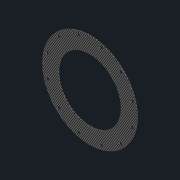
# Autodesk Inventor part: unit-plate3
Saved by Autodesk Inventor 2021 (Build 250183000, 183)
## iProperties
Created: 2021-07-12
Part Number: unit-plate3
Material: CFRP
Document SubType Name: Sheet Metal
Designer: yuta0
Density: 1.43 g/cm^3
Sheet Metal Rule: Default_mm
Appearance: カーボンファイバー
Mass: 9.12373 g
Surface Area: 136.539 cm^2
Volume: 6.38023 cm^3
Author: yuta0
Autodesk Inventor part; units mm, degrees
ref_plane "YZ Plane" through (0, 0, 0) normal (1, 0, 0) x (0, 1, 0)
ref_plane "XZ Plane" through (0, 0, 0) normal (0, 1, 0) x (-1, 0, 0)
ref_plane "XY Plane" through (0, 0, 0) normal (0, 0, 1) x (1, 0, 0)
sketch "スケッチ4" plane through (0, 0, 1) normal (0, 0, 1) x (1, 0, 0)
  circle A0 centre (16.1762, 60.3704) radius 2.25 projected
  circle A1 centre (-16.1762, 60.3704) radius 2.25 projected
  circle A2 centre (0, 0) radius 67.5 projected
  circle A3 centre (-16.1762, 60.3704) radius 5
  circle A4 centre (16.1762, 60.3704) radius 5
  circle A5 centre (0, 0) radius 62.5
  point P0 (-11.2987, 61.4702)
  point P1 (11.2987, 61.4702)
  point P2 (17.4703, 65.2)
  point P3 (-17.4703, 65.2)
  constraints: 2 centre point, 2 tangent, 3 other
sketch "スケッチ1" plane through (0, 0, 0) normal (0, 0, 1) x (1, 0, 0)
  circle A0 centre (0, 0) radius 67.5
  dimension "d0" = 135
  measures "d0" diameter of A0
extrude "プレート1" add sketch "スケッチ1" along normal blind 1
sketch "スケッチ2" plane through (0, 0, 1) normal (0, 0, 1) x (1, 0, 0)
  circle A0 centre (0, 0) radius 44.5
  dimension "d2" = 89
  constraints: 1 centre point, 1 coincident
  measures "d2" diameter of A0
extrude "押し出し1" cut sketch "スケッチ2" against normal through all
sketch "スケッチ3" plane through (0, 0, 1) normal (0, 0, 1) x (1, 0, 0)
  circle A0 centre (0, 0) radius 62.5
  point P0 (16.1762, 60.3704)
  point P1 (-16.1762, 60.3704)
  point P2 (-44.1942, 44.1942)
  point P3 (-60.3704, 16.1762)
  point P4 (-60.3704, -16.1762)
  point P5 (-44.1942, -44.1942)
  point P6 (-16.1762, -60.3704)
  point P7 (16.1762, -60.3704)
  point P8 (44.1942, -44.1942)
  point P9 (60.3704, -16.1762)
  point P10 (60.3704, 16.1762)
  point P11 (44.1942, 44.1942)
  dimension "d5" = 125
  dimension "d8" = 360
  dimension "d23" = 0
  constraints: 1 coincident, 16 other
  measures "d23" vertical distance of point (-16.176, 60.37) point (16.176, 60.37)
hole "穴1" at (16.1762, 60.3704, 1) at (-16.1762, 60.3704, 1) at (-44.1942, 44.1942, 1) at (-60.3704, 16.1762, 1) at (-60.3704, -16.1762, 1) at (-44.1942, -44.1942, 1) at (-16.1762, -60.3704, 1) at (16.1762, -60.3704, 1) at (44.1942, -44.1942, 1) at (60.3704, -16.1762, 1) at (60.3704, 16.1762, 1) at (44.1942, 44.1942, 1) direction (0, 0, -1) diameter 4.5 end through all clearance for "Flat Head Machine Screw" size "M4" standard "Ansi Metric M Profile"
equation "\"d15\" = Thickness"
equation "\"d1\" = Thickness"
equation "\"BendRadius\" = Thickness"
equation "\"BendReliefWidth\" = Thickness"
equation "\"BendReliefDepth\" = 0.5 * Thickness"
equation "\"CornerReliefSize\" = 4 * Thickness"
equation "\"MinimumRemnant\" = 2 * Thickness"
equation "\"TransitionRadius\" = BendRadius"
equation "\"JacobiRadiusSize\" = BendRadius"
equation "\"GapSize\" = Thickness"
equation "\"Thickness\" = 1"
